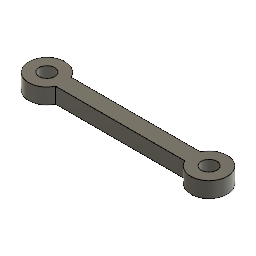
elo v1 (Autodesk Fusion 360 design; units mm, degrees)
Autodesk Fusion 360 part; units mm, degrees
note: some values were not read from the file. Set by a fixed rule: which sketch regions a step uses.
sketch "Sketch1" plane through (0, 0, 0) normal (0, 1, 0) x (1, 0, 0)
  circle A0 centre (0, 0) radius 3.5
  circle A1 centre (0, 0) radius 1.5
  circle A2 centre (31, 0) radius 1.5
  circle A3 centre (31, 0) radius 3.5
  line L0 (0, 0) -> (31, 0)
  line L1 (3.1623, 1.5) -> (27.8377, 1.5)
  line L2 (3.1623, -1.5) -> (27.8377, -1.5)
  dimension "d1" = 3
  dimension "d2" = 7
  dimension "d3" = 3
  dimension "d4" = 7
  dimension "d5" = 31
  dimension "d6" = 1.5
  dimension "d7" = 1.5
  constraint coincident A0.centre A1.centre
  constraint concentric A2 A3
  constraint coincident A2.centre A3.centre
  constraint horizontal L0
  constraint coincident A0 L1.start
  constraint coincident A3 L1.end
  constraint horizontal L1
  constraint coincident A0 L2.start
  constraint coincident A3 L2.end
  constraint horizontal L2
  measures "d1" diameter of A1
  measures "d2" diameter of A0
  measures "d3" diameter of A2
  measures "d4" diameter of A3
  measures "d5" distance of A0.centre A2.centre
  measures "d6" distance of L0 L1
  measures "d7" distance of L0 L2
extrude "Extrude1" add sketch "Sketch1" along normal blind 3
